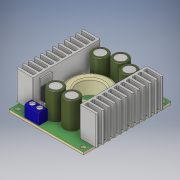
# Autodesk Inventor part: DC-DC sown
Saved by Autodesk Inventor 2019 (Build 230136000, 136)
## iProperties
Created: 2020-12-31
Part Number: DC-DC sown
Material: Типовые
Document SubType Name: Modeling
Designer: Professional
Density: 1 g/cm^3
Appearance: По умолчанию
Author: Professional
Autodesk Inventor part; units mm, degrees
ref_plane "YZ Plane" through (0, 0, 0) normal (1, 0, 0) x (0, 1, 0)
ref_plane "XZ Plane" through (0, 0, 0) normal (0, 1, 0) x (-1, 0, 0)
ref_plane "XY Plane" through (0, 0, 0) normal (0, 0, 1) x (1, 0, 0)
sketch "Эскиз1" plane through (0, 0, 0) normal (0, 1, 0) x (-1, 0, 0)
  line L0 (25.5, 30) -> (-25.5, 30)
  line L1 (-25.5, 30) -> (-25.5, -30)
  line L2 (-25.5, -30) -> (25.5, -30)
  line L3 (25.5, -30) -> (25.5, 30)
  point P0 (0, 0)
  point P1 (0, 30)
  point P2 (-25.5, 0)
  dimension "d0" = 60
  dimension "d1" = 51
  constraints: 8 end point, 2 midpoint, 2 parallel, 1 horizontal, 1 horizontal alignment, 1 perpendicular, 1 vertical alignment
  measures "d0" distance of L0.end L1.end
  measures "d1" distance between parallel lines of L1 L3
extrude "Выдавливание1" add sketch "Эскиз1" along normal blind 1.6
sketch "Эскиз2" plane through (0, 1.6, 0) normal (0, 1, 0) x (1, 0, 0)
  line L0 (25.5, -30) -> (25.5, 30) projected
  line L1 (25.5, 0) -> (-25.5, 0)
  line L2 (-25.5, 30) -> (-25.5, -30) projected
  line L3 (-25.5, -30) -> (25.5, -30) projected
  line L4 (0, -30) -> (0, 30)
  line L5 (25.5, 30) -> (-25.5, 30) projected
  point P0 (0, 0)
  point P1 (-22.5, -27)
  point P2 (-22.5, 27)
  point P3 (22.5, 27)
  point P4 (22.5, -27)
  dimension "d11" = 3
  dimension "d12" = 3
  constraints: 4 end point, 4 midpoint, 4 symmetric about line
  measures "d11" distance from line of L5 point (-22.5, 27)
  measures "d12" distance from line of L2 point (-22.5, 27)
hole "Отверстие1" at (-22.5, 1.6, 27) at (-22.5, 1.6, -27) at (22.5, 1.6, -27) at (22.5, 1.6, 27) direction (0, -1, 0) diameter 3 end through all
sketch "Эскиз3" plane through (0, 1.6, 0) normal (0, 1, 0) x (1, 0, 0)
  line L0 (15.9, -23) -> (17.5, -23)
  line L1 (17.5, -23) -> (17.5, 23)
  line L2 (17.5, 23) -> (15.9, 23)
  line L3 (15.9, 23) -> (15.9, -23)
  line L4 (17.5, -23) -> (27.5, -23)
  line L5 (27.5, -23) -> (27.5, -21.4)
  line L6 (27.5, -21.4) -> (17.5, -21.4)
  line L7 (17.5, -21.4) -> (17.5, -23)
  line L8 (25.5, -30) -> (25.5, 30) projected
  line L9 (25.5, 0) -> (-25.5, 0) construction
  line L10 (-25.5, 30) -> (-25.5, -30) projected
  line L11 (17.5, -19) -> (27.5, -19)
  line L12 (27.5, -19) -> (27.5, -17.4)
  line L13 (27.5, -17.4) -> (17.5, -17.4)
  line L14 (17.5, -17.4) -> (17.5, -19)
  line L15 (17.5, -15) -> (27.5, -15)
  line L16 (27.5, -15) -> (27.5, -13.4)
  line L17 (27.5, -13.4) -> (17.5, -13.4)
  line L18 (17.5, -13.4) -> (17.5, -15)
  line L19 (17.5, -11) -> (27.5, -11)
  line L20 (27.5, -11) -> (27.5, -9.4)
  line L21 (27.5, -9.4) -> (17.5, -9.4)
  line L22 (17.5, -9.4) -> (17.5, -11)
  line L23 (17.5, -7) -> (27.5, -7)
  line L24 (27.5, -7) -> (27.5, -5.4)
  line L25 (27.5, -5.4) -> (17.5, -5.4)
  line L26 (17.5, -5.4) -> (17.5, -7)
  line L27 (17.5, -3) -> (27.5, -3)
  line L28 (27.5, -3) -> (27.5, -1.4)
  line L29 (27.5, -1.4) -> (17.5, -1.4)
  line L30 (17.5, -1.4) -> (17.5, -3)
  line L31 (17.5, 23) -> (27.5, 23)
  line L32 (27.5, 23) -> (27.5, 21.4)
  line L33 (27.5, 21.4) -> (17.5, 21.4)
  line L34 (17.5, 21.4) -> (17.5, 23)
  line L35 (17.5, 19) -> (27.5, 19)
  line L36 (27.5, 19) -> (27.5, 17.4)
  line L37 (27.5, 17.4) -> (17.5, 17.4)
  line L38 (17.5, 17.4) -> (17.5, 19)
  line L39 (17.5, 15) -> (27.5, 15)
  line L40 (27.5, 15) -> (27.5, 13.4)
  line L41 (27.5, 13.4) -> (17.5, 13.4)
  line L42 (17.5, 13.4) -> (17.5, 15)
  line L43 (17.5, 11) -> (27.5, 11)
  line L44 (27.5, 11) -> (27.5, 9.4)
  line L45 (27.5, 9.4) -> (17.5, 9.4)
  line L46 (17.5, 9.4) -> (17.5, 11)
  line L47 (17.5, 7) -> (27.5, 7)
  line L48 (27.5, 7) -> (27.5, 5.4)
  line L49 (27.5, 5.4) -> (17.5, 5.4)
  line L50 (17.5, 5.4) -> (17.5, 7)
  line L51 (17.5, 3) -> (27.5, 3)
  line L52 (27.5, 3) -> (27.5, 1.4)
  line L53 (27.5, 1.4) -> (17.5, 1.4)
  line L54 (17.5, 1.4) -> (17.5, 3)
  line L55 (0, -30) -> (0, 30) construction
  line L56 (25.5, 30) -> (-25.5, 30) projected
  line L57 (-25.5, -30) -> (25.5, -30) construction
  line L58 (-15.9, -23) -> (-17.5, -23)
  line L59 (-17.5, -23) -> (-17.5, 23)
  line L60 (-17.5, 23) -> (-15.9, 23)
  line L61 (-15.9, 23) -> (-15.9, -23)
  line L62 (-17.5, -23) -> (-27.5, -23)
  line L63 (-27.5, -23) -> (-27.5, -21.4)
  line L64 (-27.5, -21.4) -> (-17.5, -21.4)
  line L65 (-17.5, -21.4) -> (-17.5, -23)
  line L66 (-25.5, -30) -> (-25.5, 30)
  line L67 (-25.5, 0) -> (25.5, 0)
  line L68 (-17.5, -19) -> (-27.5, -19)
  line L69 (-27.5, -19) -> (-27.5, -17.4)
  line L70 (-27.5, -17.4) -> (-17.5, -17.4)
  line L71 (-17.5, -17.4) -> (-17.5, -19)
  line L72 (-17.5, -15) -> (-27.5, -15)
  line L73 (-27.5, -15) -> (-27.5, -13.4)
  line L74 (-27.5, -13.4) -> (-17.5, -13.4)
  line L75 (-17.5, -13.4) -> (-17.5, -15)
  line L76 (-17.5, -11) -> (-27.5, -11)
  line L77 (-27.5, -11) -> (-27.5, -9.4)
  line L78 (-27.5, -9.4) -> (-17.5, -9.4)
  line L79 (-17.5, -9.4) -> (-17.5, -11)
  line L80 (-17.5, -7) -> (-27.5, -7)
  line L81 (-27.5, -7) -> (-27.5, -5.4)
  line L82 (-27.5, -5.4) -> (-17.5, -5.4)
  line L83 (-17.5, -5.4) -> (-17.5, -7)
  line L84 (-17.5, -3) -> (-27.5, -3)
  line L85 (-27.5, -3) -> (-27.5, -1.4)
  line L86 (-27.5, -1.4) -> (-17.5, -1.4)
  line L87 (-17.5, -1.4) -> (-17.5, -3)
  line L88 (-17.5, 9.4) -> (-17.5, 11)
  line L89 (-17.5, 5.4) -> (-17.5, 7)
  line L90 (-17.5, 1.4) -> (-17.5, 3)
  line L91 (-17.5, 11) -> (-27.5, 11)
  line L92 (-27.5, 11) -> (-27.5, 9.4)
  line L93 (-27.5, 9.4) -> (-17.5, 9.4)
  line L94 (-27.5, 1.4) -> (-17.5, 1.4)
  line L95 (-27.5, 3) -> (-27.5, 1.4)
  line L96 (-17.5, 3) -> (-27.5, 3)
  line L97 (-27.5, 7) -> (-27.5, 5.4)
  line L98 (-27.5, 5.4) -> (-17.5, 5.4)
  line L99 (-17.5, 7) -> (-27.5, 7)
  line L100 (-17.5, 21.4) -> (-17.5, 23)
  line L101 (-17.5, 23) -> (-27.5, 23)
  line L102 (-27.5, 23) -> (-27.5, 21.4)
  line L103 (-27.5, 21.4) -> (-17.5, 21.4)
  line L104 (-17.5, 19) -> (-27.5, 19)
  line L105 (-27.5, 19) -> (-27.5, 17.4)
  line L106 (-27.5, 17.4) -> (-17.5, 17.4)
  line L107 (-27.5, 15) -> (-27.5, 13.4)
  line L108 (-27.5, 13.4) -> (-17.5, 13.4)
  line L109 (-17.5, 15) -> (-27.5, 15)
  line L110 (-17.5, 13.4) -> (-17.5, 15)
  line L111 (-17.5, 17.4) -> (-17.5, 19)
  point P0 (0, 0)
  dimension "d13" = 1.6
  dimension "d14" = 46
  dimension "d15" = 10
  dimension "d16" = 2
  dimension "d19" = 4
  constraints: 216 end point, 75 symmetric about line, 4 midpoint, 4 parallel, 3 horizontal, 3 perpendicular, 2 vertical, 41 other
  measures "d13" distance between parallel lines of L3 L1
  measures "d14" distance between parallel lines of L2 L0
  measures "d15" distance between parallel lines of L5 L1
  measures "d16" distance between parallel lines of L8 L5
  measures "d19" distance of L0.end L11.start
extrude "Выдавливание2" add sketch "Эскиз3" along normal blind 20 contours L3 L67 L1 L0 | L1 L6 L8 L4 | L3 L2 L1 L67 | L8 L6 L5 L4 | L67 L59 L60 L61 | L61 L58 L59 L67 | L1 L13 L8 L11 | L31 L8 L33 L1 | L29 L8 L27 L1 | L1 L51 L8 L53 | L8 L13 L12 L11 | L31 L32 L33 L8 | L59 L103 L10 L101 | L62 L10 L64 L59 | L59 L84 L10 L86 | L94 L10 L96 L59 | L29 L28 L27 L8 | L8 L51 L52 L53 | L1 L17 L8 L15 | L35 L8 L37 L1 | L10 L103 L102 L101 | L62 L63 L64 L10 | L10 L84 L85 L86 | L94 L95 L96 L10 | L25 L8 L23 L1 | L1 L47 L8 L49 | L8 L17 L16 L15 | L35 L36 L37 L8 | L59 L106 L10 L104 | L68 L10 L70 L59 | L59 L80 L10 L82 | L98 L10 L99 L59 | L25 L24 L23 L8 | L8 L47 L48 L49 | L1 L21 L8 L19 | L39 L8 L41 L1 | L10 L106 L105 L104 | L68 L69 L70 L10 | L10 L80 L81 L82 | L98 L97 L99 L10 | L1 L43 L8 L45 | L8 L21 L20 L19 | L39 L40 L41 L8 | L59 L108 L10 L109 | L72 L10 L74 L59 | L59 L76 L10 L78 | L93 L10 L91 L59 | L8 L43 L44 L45 | L10 L108 L107 L109 | L72 L73 L74 L10 | L10 L76 L77 L78 | L93 L92 L91 L10
sketch "Эскиз4" plane through (0, 1.6, 0) normal (0, 1, 0) x (1, 0, 0)
  circle A0 centre (0, 0) radius 13.5
  circle A1 centre (0, 0) radius 8.5
  dimension "d26" = 5
  dimension "d27" = 17
  constraints: 2 centre point, 2 coincident
  measures "d26" radial gap between concentric circles of A0 A1
  measures "d27" diameter of A1
extrude "Выдавливание3" add sketch "Эскиз4" along normal blind 10
fillet "Сопряжение1" radius 1 2 edges at (-13.5, 11.6, 0) (-8.5, 11.6, 0)
sketch "Эскиз5" plane through (0, 1.6, 0) normal (0, 1, 0) x (1, 0, 0)
  circle A0 centre (10, 17) radius 5
  circle A1 centre (0, 21) radius 5
  circle A2 centre (-10, 17) radius 5
  circle A3 centre (5.5, -18) radius 5
  circle A4 centre (-5.5, -18) radius 5
  line L0 (25.5, 30) -> (-25.5, 30) projected
  line L1 (0, 30) -> (0, -30)
  line L2 (-25.5, -30) -> (25.5, -30) projected
  point P0 (0, 0)
  dimension "d31" = 10
  dimension "d32" = 20
  dimension "d33" = 4
  dimension "d34" = 13
  dimension "d35" = 11
  dimension "d36" = 12
  constraints: 5 centre point, 4 equal radius, 2 end point, 2 midpoint, 1 point on line, 2 other
  measures "d31" diameter of A1
  measures "d32" distance of A2.centre A0.centre
  measures "d33" vertical distance of A2.centre A1.centre
  measures "d34" distance from line of L0 A2.centre
  measures "d35" distance of A3.centre A4.centre
  measures "d36" distance from line of L2 A4.centre
extrude "Выдавливание4" add sketch "Эскиз5" along normal blind 18
sketch "Эскиз6" plane through (5.5, 19.6, 18) normal (0, 1, 0) x (1, 0, 0)
  circle A0 centre (0, 0) radius 5 projected
  circle A1 centre (-11, 0) radius 5 projected
  circle A2 centre (-15.5, 35) radius 5 projected
  circle A3 centre (-5.5, 39) radius 5 projected
  circle A4 centre (4.5, 35) radius 5 projected
  circle A5 centre (4.5, 35) radius 3.5
  circle A6 centre (-5.5, 39) radius 3.5
  circle A7 centre (-15.5, 35) radius 3.5
  circle A8 centre (-11, 0) radius 3.5
  circle A9 centre (0, 0) radius 3.5
  point P0 (-5.5, 18)
  dimension "d39" = 7
  constraints: 5 centre point, 5 coincident, 4 equal radius
  measures "d39" diameter of A9
extrude "Выдавливание5" cut sketch "Эскиз6" against normal blind 0.2 contours A5 | A6 | A7 | A8 | A9
sketch "Эскиз8" plane through (15.9, 1.6, -23) normal (-1, 0, 0) x (0, 0, 1)
  line L0 (42, 18) -> (34, 18)
  line L1 (34, 18) -> (34, 5)
  line L2 (34, 5) -> (42, 5)
  line L3 (42, 5) -> (42, 18)
  line L4 (46, 0) -> (46, 20) projected
  line L5 (0, 20) -> (46, 20) projected
  point P0 (23, -1.6)
  dimension "d43" = 8
  dimension "d44" = 13
  dimension "d45" = 4
  dimension "d46" = 2
  constraints: 8 end point, 2 parallel, 1 horizontal, 1 perpendicular
  measures "d43" distance between parallel lines of L3 L1
  measures "d44" distance between parallel lines of L0 L2
  measures "d45" distance between parallel lines of L4 L3
  measures "d46" distance between parallel lines of L5 L0
extrude "Выдавливание6" add sketch "Эскиз8" along normal blind 1
sketch "Эскиз9" plane through (14.9, 1.6, -23) normal (-1, 0, 0) x (0, 0, 1)
  line L0 (42, 5) -> (34, 5) construction
  line L1 (46, 0) -> (0, 0) construction
  line L2 (35.9, 5) -> (34.9, 5)
  line L3 (34.9, 5) -> (34.9, 0)
  line L4 (34.9, 0) -> (35.9, 0)
  line L5 (35.9, 0) -> (35.9, 5)
  line L6 (37.5, 5) -> (38.5, 5)
  line L7 (38.5, 5) -> (38.5, 0)
  line L8 (38.5, 0) -> (37.5, 0)
  line L9 (37.5, 0) -> (37.5, 5)
  line L10 (41.1, 5) -> (40.1, 5)
  line L11 (40.1, 5) -> (40.1, 0)
  line L12 (40.1, 0) -> (41.1, 0)
  line L13 (41.1, 0) -> (41.1, 5)
  line L14 (34, 18) -> (42, 18) projected
  line L15 (38, 18) -> (38, -1.6)
  line L16 (53, -1.6) -> (-7, -1.6) projected
  point P0 (23, -1.6)
  dimension "d49" = 1
  dimension "d50" = 1.6
  constraints: 26 end point, 7 point on line, 6 parallel, 3 horizontal, 3 perpendicular, 1 collinear, 1 midpoint, 1 vertical, 3 other
  measures "d49" distance between parallel lines of L13 L11
  measures "d50" distance between parallel lines of L7 L11
extrude "Выдавливание7" add sketch "Эскиз9" along normal blind 0.4
sketch "Эскиз10" plane through (14.9, 1.6, -23) normal (-1, 0, 0) x (0, 0, 1)
  line L0 (34.05, 5.1) -> (41.95, 5.1)
  line L1 (41.95, 5.1) -> (41.95, 13)
  line L2 (41.95, 13) -> (34.05, 13)
  line L3 (34.05, 13) -> (34.05, 5.1)
  line L4 (34, 18) -> (42, 18) projected
  line L5 (42, 5) -> (34, 5) projected
  point P0 (23, -1.6)
  point P1 (38, 13)
  point P2 (38, 18)
  dimension "d74" = 7.9
  dimension "d75" = 0.1
  dimension "d76" = 5
  constraints: 8 end point, 2 midpoint, 2 parallel, 1 horizontal, 1 perpendicular, 1 vertical alignment
  measures "d74" distance between parallel lines of L1 L3
  measures "d75" distance between parallel lines of L0 L5
  measures "d76" distance between parallel lines of L4 L2
extrude "Выдавливание8" add sketch "Эскиз10" along normal blind 3
fillet "Сопряжение2" radius 0.5 48 edges at (27.5, 11.6, 9.4) (27.5, 11.6, 11) (27.5, 11.6, 13.4) (27.5, 11.6, 15) (27.5, 11.6, 17.4) (27.5, 11.6, 19) (27.5, 11.6, 21.4) (27.5, 11.6, 23) (27.5, 11.6, 7) (27.5, 11.6, 5.4) (27.5, 11.6, 3) (27.5, 11.6, 1.4) (27.5, 11.6, -1.4) (27.5, 11.6, -3) (27.5, 11.6, -5.4) (27.5, 11.6, -7) (27.5, 11.6, -9.4) (27.5, 11.6, -11) (27.5, 11.6, -13.4) (27.5, 11.6, -15) (27.5, 11.6, -17.4) (27.5, 11.6, -19) (27.5, 11.6, -21.4) (27.5, 11.6, -23) (17.5, 11.6, -3) (17.5, 11.6, -5.4) (17.5, 11.6, -9.4) (17.5, 11.6, -1.4) (17.5, 11.6, 3) (17.5, 11.6, 7) (17.5, 11.6, 11) (17.5, 11.6, 15) (17.5, 11.6, 19) (17.5, 11.6, -13.4) (17.5, 11.6, -17.4) (17.5, 11.6, -21.4) (17.5, 11.6, -19) (17.5, 11.6, -15) (17.5, 11.6, -11) (17.5, 11.6, -7) (17.5, 11.6, 1.4) (17.5, 11.6, 5.4) (17.5, 11.6, 9.4) (17.5, 11.6, 13.4) (17.5, 11.6, 17.4) (17.5, 11.6, 21.4) (15.9, 11.6, -23) (15.9, 11.6, 23)
mirror "Зеркальное отражение1" about plane through (0, 0, 0) normal (1, 0, 0) of "Выдавливание6", "Выдавливание7", "Выдавливание8", "Сопряжение2"
fillet "Сопряжение3" radius 0.5 5 edges at (-10.5, 19.6, 18) (0.5, 19.6, 18) (5, 19.6, -17) (-5, 19.6, -21) (-15, 19.6, -17)
sketch "Эскиз11" plane through (0, 1.6, 0) normal (0, 1, 0) x (1, 0, 0)
  line L0 (-15.5, -29.5) -> (-5.5, -29.5)
  line L1 (-5.5, -29.5) -> (-5.5, -23.5)
  line L2 (-5.5, -23.5) -> (-15.5, -23.5)
  line L3 (-15.5, -23.5) -> (-15.5, -29.5)
  line L4 (17.5, 29.5) -> (7.5, 29.5)
  line L5 (7.5, 29.5) -> (7.5, 23.5)
  line L6 (7.5, 23.5) -> (17.5, 23.5)
  line L7 (17.5, 23.5) -> (17.5, 29.5)
  line L8 (25.5, 30) -> (-25.5, 30) projected
  line L9 (25.5, 23) -> (25.5, 30) projected
  line L10 (-25.5, -30) -> (25.5, -30) projected
  line L11 (-25.5, -23) -> (-25.5, -30) projected
  point P0 (0, 0)
  dimension "d58" = 10
  dimension "d59" = 6
  dimension "d60" = 0.5
  dimension "d61" = 8
  dimension "d62" = 0.5
  dimension "d63" = 10
  constraints: 16 end point, 6 parallel, 2 horizontal, 2 perpendicular
  measures "d58" distance between parallel lines of L7 L5
  measures "d59" distance between parallel lines of L4 L6
  measures "d60" distance between parallel lines of L8 L4
  measures "d61" distance between parallel lines of L9 L7
  measures "d62" distance between parallel lines of L10 L0
  measures "d63" distance between parallel lines of L11 L3
extrude "Выдавливание9" add sketch "Эскиз11" along normal blind 8
sketch "Эскиз12" plane through (0, 9.6, 0) normal (0, 1, 0) x (1, 0, 0)
  circle A0 centre (-13, -26.5) radius 1.75
  circle A1 centre (-8, -26.5) radius 1.75
  circle A2 centre (10, 26.5) radius 1.75
  circle A3 centre (15, 26.5) radius 1.75
  line L0 (17.5, 23.5) -> (17.5, 29.5) projected
  line L1 (-15.5, -23.5) -> (-15.5, -29.5) projected
  line L2 (-5.5, -29.5) -> (-15.5, -29.5) projected
  line L3 (-10.5, -29.5) -> (-10.5, -23.5)
  line L4 (-5.5, -23.5) -> (-15.5, -23.5) projected
  line L5 (17.5, 23.5) -> (7.5, 23.5) projected
  line L6 (12.5, 23.5) -> (12.5, 29.5)
  line L7 (17.5, 29.5) -> (7.5, 29.5) projected
  point P0 (0, 0)
  point P1 (17.5, 26.5)
  point P2 (-15.5, -26.5)
  dimension "d66" = 3.5
  dimension "d67" = 5
  dimension "d68" = 5
  constraints: 6 midpoint, 4 centre point, 4 end point, 4 horizontal alignment, 3 equal radius, 2 other
  measures "d66" diameter of A3
  measures "d67" distance of A3.centre A2.centre
  measures "d68" distance of A1.centre A0.centre
extrude "Выдавливание10" cut sketch "Эскиз12" against normal blind 1 contours A0 | A1 | A2 | A3
chamfer "Фаска1" distance 1 angle 45 4 edges at (-10.5, 9.6, 29.5) (-10.5, 9.6, 23.5) (12.5, 9.6, -23.5) (12.5, 9.6, -29.5)
